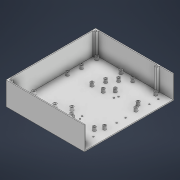
# Autodesk Inventor part: Grundplatte_vorne
Saved by Autodesk Inventor 2021 (Build 250183000, 183)
## iProperties
Created: 2021-01-26
Part Number: Grundplatte_vorne
Material: Generisch
Document SubType Name: Modeling
Designer: Ctroi
Density: 1 g/cm^3
Appearance: Vorgabe
Author: Ctroi
Autodesk Inventor part; units mm, degrees
ref_plane "YZ Plane" through (0, 0, 0) normal (1, 0, 0) x (0, 1, 0)
ref_plane "XZ Plane" through (0, 0, 0) normal (0, 1, 0) x (-1, 0, 0)
ref_plane "XY Plane" through (0, 0, 0) normal (0, 0, 1) x (1, 0, 0)
sketch "Skizze1" plane through (0, 0, 0) normal (0, 1, 0) x (-1, 0, 0)
  line L0 (0, -140) -> (0, 140) projected
  line L1 (-122.5, 0) -> (122.5, 0) projected
  line L2 (87.5, -100) -> (-87.5, -100)
  line L3 (-87.5, -100) -> (-87.5, 100)
  line L4 (-87.5, 100) -> (87.5, 100)
  line L5 (87.5, 100) -> (87.5, -100)
  point P0 (0, 0)
  dimension "d0" = 175
  dimension "d1" = 200
  constraints: 8 end point, 2 parallel, 1 horizontal, 1 perpendicular, 2 other
  measures "d0" distance of L3.end L4.end
  measures "d1" distance of L2.end L3.end
extrude "Extrusion1" add sketch "Skizze1" along normal blind 2
sketch "Skizze2" plane through (0, 2, 0) normal (0, 1, 0) x (1, 0, 0)
  circle A0 centre (70, 82.5) radius 1.6
  line L0 (87.5, -100) -> (87.5, 100) projected
  line L1 (87.5, 100) -> (-87.5, 100) projected
  circle A1 centre (70, 62.5) radius 1.6
  line L2 (122.5, 0) -> (-122.5, 0) projected
  circle A2 centre (70, -82.5) radius 1.6
  circle A3 centre (70, -62.5) radius 1.6
  point P0 (0, 0)
  dimension "d4" = 3.2
  dimension "d5" = 17.5
  dimension "d6" = 17.5
  dimension "d7" = 3.2
  dimension "d8" = 20
  dimension "d9" = 17.5
  constraints: 4 centre point, 2 symmetric about line, 2 other
  measures "d4" diameter of A0
  measures "d5" distance from line of L0 A0.centre
  measures "d6" distance from line of L1 A0.centre
  measures "d7" diameter of A1
  measures "d8" distance of A0.centre A1.centre
  measures "d9" distance from line of L0 A1.centre
extrude "Extrusion2" cut sketch "Skizze2" against normal up to surface (2 mm away)
sketch "Skizze4" plane through (0, 2, 0) normal (0, 1, 0) x (1, 0, 0)
  line L0 (-87.5, -100) -> (87.5, -100) projected
  line L1 (-87.5, 100) -> (-87.5, -100) projected
  line L2 (87.5, -100) -> (-87.5, -100)
  line L3 (-87.5, -100) -> (-87.5, -98)
  line L4 (-87.5, -98) -> (87.5, -98)
  line L5 (87.5, -98) -> (87.5, -100)
  line L6 (87.5, 100) -> (-87.5, 100) projected
  line L7 (87.5, 100) -> (-87.5, 100)
  line L8 (-87.5, 100) -> (-87.5, 98)
  line L9 (-87.5, 98) -> (87.5, 98)
  line L10 (87.5, 98) -> (87.5, 100)
  line L11 (87.5, -98) -> (51.5, -98)
  line L12 (51.5, -98) -> (51.5, -92)
  line L13 (51.5, -92) -> (57.5, -92)
  line L14 (87.5, 98) -> (51.5, 98)
  line L15 (51.5, 98) -> (51.5, 92)
  line L16 (51.5, 92) -> (57.5, 92)
  line L17 (-87.5, -98) -> (-85.5, -98)
  line L18 (-85.5, -98) -> (-85.5, 98)
  line L19 (-85.5, 98) -> (-87.5, 98)
  line L20 (-87.5, 98) -> (-87.5, -98)
  line L21 (-85.5, 98) -> (-79.5, 98)
  line L22 (-79.5, 98) -> (-79.5, 92)
  line L23 (-79.5, 92) -> (-85.5, 92)
  line L24 (-85.5, 92) -> (-85.5, 98)
  line L25 (-85.5, -98) -> (-79.5, -98)
  line L26 (-79.5, -98) -> (-79.5, -92)
  line L27 (-79.5, -92) -> (-85.5, -92)
  line L28 (-85.5, -92) -> (-85.5, -98)
  line L29 (57.5, -92) -> (57.5, -98)
  line L30 (87.5, -100) -> (87.5, 100) projected
  line L31 (57.5, 98) -> (57.5, 92)
  point P0 (0, 0)
  point P1 (-85.5, -92)
  point P2 (51.5, -98)
  point P3 (-87.5, 98)
  point P4 (-87.5, 100)
  dimension "d18" = 2
  dimension "d19" = 2
  dimension "d21" = 6
  dimension "d23" = 6
  dimension "d24" = 2
  dimension "d25" = 6
  dimension "d26" = 6
  dimension "d27" = 6
  dimension "d28" = 6
  dimension "d130" = 6
  dimension "d131" = 30
  dimension "d132" = 6
  dimension "d133" = 30
  constraints: 56 end point, 12 parallel, 9 perpendicular, 7 horizontal, 5 point on line
  measures "d18" distance of L2.end L3.end
  measures "d19" distance of L8.end L7.end
  measures "d21" distance of L11.end L12.end
  measures "d23" distance of L15.end L14.end
  measures "d24" distance of L19.end L18.end
  measures "d25" distance of L22.end L23.end
  measures "d26" distance of L21.end L22.end
  measures "d27" distance of L27.end L26.end
  measures "d28" distance of L26.end L25.end
  measures "d130" distance between parallel lines of L12 L29
  measures "d131" distance between parallel lines of L30 L29
  measures "d132" distance between parallel lines of L31 L15
  measures "d133" distance between parallel lines of L30 L31
extrude "Extrusion4" add sketch "Skizze4" along normal blind 50 contours L1 L4 L5 L0 | L1 L9 L18 L4 | L1 L6 L10 L9 | L18 L27 L26 L4 | L4 L12 L13 L29 | L9 L22 L23 L18 | L31 L16 L15 L9
sketch "Skizze5" plane through (0, 2, 0) normal (0, 1, 0) x (1, 0, 0)
  circle A0 centre (67.5, 35) radius 3.5
  circle A1 centre (67.5, -35) radius 3.5
  line L0 (-129.052, 0) -> (123.592, 0) projected
  line L1 (123.592, 0) -> (-129.052, 0) projected
  line L2 (87.5, -98) -> (87.5, 98) projected
  circle A2 centre (-5.5, -35) radius 3.5
  circle A3 centre (-5.5, 35) radius 3.5
  line L3 (87.5, 100) -> (-87.5, 100) projected
  circle A4 centre (-30, -48.325) radius 3.5
  circle A5 centre (-30, 34.225) radius 3.5
  circle A6 centre (-78.26, 27.875) radius 3.5
  circle A7 centre (-78.26, -47.055) radius 3.5
  line L4 (-87.5, 100) -> (-87.5, -100) projected
  line L5 (51.5, -98) -> (-79.5, -98) projected
  line L6 (-85.5, -92) -> (-85.5, 92) projected
  line L7 (0, 140) -> (0, -140) projected
  circle A8 centre (7.5, 49) radius 3.5
  circle A9 centre (7.5, 88) radius 3.5
  circle A10 centre (58.5, 49) radius 3.5
  circle A11 centre (58.5, 88) radius 3.5
  line L8 (-79.5, 98) -> (51.5, 98) projected
  circle A12 centre (7.5, -49) radius 3.5
  circle A13 centre (7.5, -88) radius 3.5
  circle A14 centre (58.5, -49) radius 3.5
  circle A15 centre (58.5, -88) radius 3.5
  circle A16 centre (-75.5, 56.5) radius 3.5
  circle A17 centre (-75.5, 90.5) radius 3.5
  circle A18 centre (-21.5, 56.5) radius 3.5
  circle A19 centre (-21.5, 90.5) radius 3.5
  circle A20 centre (-9, 73) radius 3.5
  circle A21 centre (-9, -73) radius 3.5
  point P0 (0, 0)
  point P1 (-75, 100)
  dimension "d31" = 7
  dimension "d32" = 7
  dimension "d35" = 20
  dimension "d36" = 20
  dimension "d37" = 7
  dimension "d38" = 73
  dimension "d40" = 7
  dimension "d42" = 73
  dimension "d68" = 70
  dimension "d69" = 70
  dimension "d70" = 35
  dimension "d73" = 65
  dimension "d74" = 7
  dimension "d75" = 7
  dimension "d83" = 7
  dimension "d86" = 7
  dimension "d136" = 48.26
  dimension "d137" = 74.93
  dimension "d138" = 48.26
  dimension "d139" = 82.55
  dimension "d142" = 30
  dimension "d143" = 30
  dimension "d144" = 34.225
  dimension "d145" = 47.055
  dimension "d148" = 7
  dimension "d149" = 7
  dimension "d150" = 7
  dimension "d151" = 7
  dimension "d152" = 10
  dimension "d153" = 10
  dimension "d154" = 39
  dimension "d155" = 39
  dimension "d156" = 51
  dimension "d157" = 51
  dimension "d161" = 7.5
  dimension "d163" = 7.5
  dimension "d177" = 7
  dimension "d178" = 7
  dimension "d179" = 7
  dimension "d180" = 7
  dimension "d181" = 10
  dimension "d182" = 10
  dimension "d183" = 7.5
  dimension "d184" = 34
  dimension "d185" = 7.5
  dimension "d186" = 34
  dimension "d187" = 54
  dimension "d188" = 54
  dimension "d193" = 7
  dimension "d194" = 25
  dimension "d195" = 9
  dimension "d196" = 7
  dimension "d197" = 25
  dimension "d198" = 9
  constraints: 22 centre point, 4 symmetric about line, 5 other
  measures "d31" diameter of A0
  measures "d32" diameter of A1
  measures "d35" distance from line of L2 A0.centre
  measures "d36" distance from line of L2 A1.centre
  measures "d37" diameter of A2
  measures "d38" distance of A1.centre A2.centre
  measures "d40" diameter of A3
  measures "d42" distance of A0.centre A3.centre
  measures "d68" distance of A0.centre A1.centre
  measures "d69" distance of A3.centre A2.centre
  measures "d70" distance from line of L0 A0.centre
  measures "d73" distance from line of L3 A3.centre
  measures "d74" diameter of A4
  measures "d75" diameter of A5
  measures "d83" diameter of A6
  measures "d86" diameter of A7
  measures "d136" horizontal distance of A4.centre A7.centre
  measures "d137" distance of A6.centre A7.centre
  measures "d138" horizontal distance of A5.centre A6.centre
  measures "d139" distance of A4.centre A5.centre
  measures "d142" distance from line of L7 A4.centre
  measures "d143" distance from line of L7 A5.centre
  measures "d144" distance from line of L1 A5.centre
  measures "d145" distance from line of L1 A7.centre
  measures "d148" diameter of A8
  measures "d149" diameter of A9
  measures "d150" diameter of A10
  measures "d151" diameter of A11
  measures "d152" distance from line of L8 A11.centre
  measures "d153" distance from line of L8 A9.centre
  measures "d154" distance of A9.centre A8.centre
  measures "d155" distance of A11.centre A10.centre
  measures "d156" distance of A11.centre A9.centre
  measures "d157" distance of A8.centre A10.centre
  measures "d161" distance from line of L7 A8.centre
  measures "d163" distance from line of L7 A9.centre
  measures "d177" diameter of A16
  measures "d178" diameter of A17
  measures "d179" diameter of A18
  measures "d180" diameter of A19
  measures "d181" distance from line of L6 A16.centre
  measures "d182" distance from line of L6 A17.centre
  measures "d183" distance from line of L8 A17.centre
  measures "d184" distance of A16.centre A17.centre
  measures "d185" distance from line of L8 A19.centre
  measures "d186" distance of A19.centre A18.centre
  measures "d187" distance of A17.centre A19.centre
  measures "d188" distance of A16.centre A18.centre
  measures "d193" diameter of A20
  measures "d194" distance from line of L8 A20.centre
  measures "d195" distance from line of L7 A20.centre
  measures "d196" diameter of A21
  measures "d197" distance from line of L5 A21.centre
  measures "d198" distance from line of L7 A21.centre
extrude "Extrusion5" add sketch "Skizze5" along normal blind 7 contours A0 | A1 | A2 | A3 | A4 | A5 | A6 | A7 | A8 | A9 | A10 | A11 | A12 | A13 | A14 | A15 | A16 | A17 | A18 | A19 | A20 | A21
sketch "Skizze6" plane through (-5.5, 9, -35) normal (0, 1, 0) x (1, 0, 0)
  circle A0 centre (0, 0) radius 2
  circle A1 centre (73, 0) radius 3.5 projected
  circle A2 centre (73, 0) radius 2
  circle A3 centre (0, -70) radius 2
  circle A4 centre (0, -70) radius 3.5 projected
  circle A5 centre (73, -70) radius 3.5 projected
  circle A6 centre (73, -70) radius 2
  circle A7 centre (-72.76, -82.055) radius 2
  circle A8 centre (-72.76, -82.055) radius 3.5 projected
  circle A9 centre (-24.5, -83.325) radius 2
  circle A10 centre (-24.5, -83.325) radius 3.5 projected
  circle A11 centre (-24.5, -0.775) radius 2
  circle A12 centre (-24.5, -0.775) radius 3.5 projected
  circle A13 centre (-72.76, -7.125) radius 2
  circle A14 centre (-72.76, -7.125) radius 3.5 projected
  circle A15 centre (13, -123) radius 3.5
  circle A16 centre (13, -123) radius 3.5 projected
  circle A17 centre (13, -123) radius 2
  circle A18 centre (13, -84) radius 3.5
  circle A19 centre (13, -84) radius 3.5 projected
  circle A20 centre (13, -84) radius 2
  circle A21 centre (64, -123) radius 2
  circle A22 centre (64, -123) radius 3.5 projected
  circle A23 centre (64, -123) radius 3.5
  circle A24 centre (64, -84) radius 3.5
  circle A25 centre (64, -84) radius 3.5 projected
  circle A26 centre (64, -84) radius 2
  line L0 (128, -35) -> (-117, -35) projected
  circle A27 centre (13, 53) radius 3.5
  circle A28 centre (13, 53) radius 2
  circle A29 centre (13, 14) radius 3.5
  circle A30 centre (13, 14) radius 2
  circle A31 centre (64, 53) radius 2
  circle A32 centre (64, 53) radius 3.5
  circle A33 centre (64, 14) radius 3.5
  circle A34 centre (64, 14) radius 2
  circle A35 centre (-70, 21.5) radius 3.5 projected
  circle A36 centre (-70, 55.5) radius 3.5 projected
  circle A37 centre (-16, 55.5) radius 3.5 projected
  circle A38 centre (-16, 21.5) radius 3.5 projected
  circle A39 centre (-70, 21.5) radius 2
  circle A40 centre (-70, 55.5) radius 3.5 projected
  circle A41 centre (-70, 55.5) radius 2
  circle A42 centre (-16, 21.5) radius 3.5 projected
  circle A43 centre (-16, 21.5) radius 2
  circle A44 centre (-16, 55.5) radius 3.5 projected
  circle A45 centre (-16, 55.5) radius 2
  circle A46 centre (-3.5, -108) radius 3.5 projected
  circle A47 centre (-3.5, 38) radius 3.5 projected
  circle A48 centre (-3.5, -108) radius 2
  circle A49 centre (-3.5, 38) radius 3.5 projected
  circle A50 centre (-3.5, 38) radius 2
  point P0 (-82, -78.8303)
  point P1 (-82, -84.6297)
  point P2 (-82, -3.9003)
  point P3 (-82, -9.6997)
  dimension "d45" = 4
  dimension "d46" = 4
  dimension "d47" = 4
  dimension "d48" = 0
  dimension "d49" = 4
  dimension "d50" = 73
  dimension "d51" = 70
  dimension "d96" = 4
  dimension "d97" = 0
  dimension "d98" = 0
  dimension "d99" = 4
  dimension "d100" = 0
  dimension "d101" = 0
  dimension "d102" = 4
  dimension "d103" = 0
  dimension "d104" = 4
  dimension "d105" = 0
  dimension "d164" = 7
  dimension "d165" = 0
  dimension "d166" = 0
  dimension "d167" = 4
  dimension "d168" = 7
  dimension "d169" = 0
  dimension "d170" = 4
  dimension "d171" = 4
  dimension "d172" = 0
  dimension "d173" = 7
  dimension "d174" = 7
  dimension "d176" = 4
  dimension "d189" = 4
  dimension "d190" = 4
  dimension "d191" = 4
  dimension "d192" = 4
  dimension "d199" = 4
  dimension "d200" = 4
  constraints: 30 centre point, 13 coincident, 8 symmetric about line, 10 other
  measures "d45" diameter of A0
  measures "d46" diameter of A2
  measures "d47" diameter of A3
  measures "d48" distance of A4.centre A3.centre
  measures "d49" diameter of A6
  measures "d50" distance of A2.centre A0.centre
  measures "d51" distance of A3.centre A0.centre
  measures "d96" diameter of A7
  measures "d97" distance of point (-72.76, -82.055) A7.centre
  measures "d98" distance of point (-72.76, -82.055) A7.centre
  measures "d99" diameter of A9
  measures "d100" distance of A10.centre A9.centre
  measures "d101" distance of A10.centre A9.centre
  measures "d102" diameter of A11
  measures "d103" distance of A12.centre A11.centre
  measures "d104" diameter of A13
  measures "d105" distance of point (-72.76, -7.125) A13.centre
  measures "d164" diameter of A15
  measures "d165" distance of A16.centre A15.centre
  measures "d166" distance of A16.centre A15.centre
  measures "d167" diameter of A17
  measures "d168" diameter of A18
  measures "d169" distance of A19.centre A18.centre
  measures "d170" diameter of A20
  measures "d171" diameter of A21
  measures "d172" distance of A22.centre A21.centre
  measures "d173" diameter of A23
  measures "d174" diameter of A24
  measures "d176" diameter of A26
  measures "d189" diameter of A39
  measures "d190" diameter of A41
  measures "d191" diameter of A43
  measures "d192" diameter of A45
  measures "d199" diameter of A48
  measures "d200" diameter of A50
extrude "Extrusion6" cut sketch "Skizze6" against normal blind 5 contours A0 | A2 | A3 | A6 | A7 | A9 | A11 | A13 | A17 | A20 | A21 | A26 | A28 | A30 | A31 | A34 | A39 | A41 | A43 | A45 | A48 | A50
sketch "Skizze7" plane through (0, 52, 0) normal (0, 1, 0) x (1, 0, 0)
  circle A0 centre (54.5, -95) radius 2
  circle A1 centre (-82.5, -95) radius 2
  circle A2 centre (-82.5, 95) radius 2
  circle A3 centre (54.5, 95) radius 2
  line L0 (51.5, 98) -> (51.5, 92) projected
  line L1 (51.5, 92) -> (57.5, 92) projected
  line L2 (51.5, -92) -> (51.5, -98) projected
  line L3 (57.5, -92) -> (51.5, -92) projected
  line L4 (-79.5, -98) -> (-79.5, -92) projected
  line L5 (-79.5, -92) -> (-85.5, -92) projected
  line L6 (-79.5, 92) -> (-79.5, 98) projected
  line L7 (-85.5, 92) -> (-79.5, 92) projected
  line L8 (57.5, -98) -> (57.5, -92) projected
  line L9 (57.5, 92) -> (57.5, 98) projected
  point P0 (0, 0)
  point P1 (75, -92)
  dimension "d54" = 4
  dimension "d55" = 4
  dimension "d56" = 4
  dimension "d57" = 4
  dimension "d59" = 3
  dimension "d61" = 3
  dimension "d62" = 3
  dimension "d63" = 3
  dimension "d64" = 3
  dimension "d65" = 3
  dimension "d146" = 3
  dimension "d147" = 3
  constraints: 4 centre point
  measures "d54" diameter of A0
  measures "d55" diameter of A1
  measures "d56" diameter of A2
  measures "d57" diameter of A3
  measures "d59" distance from line of L1 A3.centre
  measures "d61" distance from line of L3 A0.centre
  measures "d62" distance from line of L4 A1.centre
  measures "d63" distance from line of L5 A1.centre
  measures "d64" distance from line of L6 A2.centre
  measures "d65" distance from line of L7 A2.centre
  measures "d146" distance from line of L2 A0.centre
  measures "d147" distance from line of L0 A3.centre
extrude "Extrusion7" cut sketch "Skizze7" against normal blind 5
sketch "Skizze8" plane through (0, 2, 0) normal (0, 1, 0) x (1, 0, 0)
  circle A0 centre (69.5, 10) radius 1.6
  line L0 (122.5, 0) -> (-122.5, 0) projected
  line L1 (87.5, -98) -> (87.5, 98) projected
  circle A1 centre (69.5, -10) radius 1.6
  circle A2 centre (20.609, 42.961) radius 1.6
  circle A3 centre (17.873, 35.444) radius 1.6
  circle A4 centre (20.609, -42.961) radius 1.6
  circle A5 centre (17.873, -35.444) radius 1.6
  point P0 (0, 0)
  point P1 (75, -92)
  point P2 (75, 92)
  point P3 (87.5, 98)
  dimension "d119" = 3.2
  dimension "d120" = 18
  dimension "d121" = 10
  dimension "d122" = 3.2
  dimension "d123" = 3.2
  dimension "d124" = 66.891
  dimension "d125" = 69.627
  dimension "d126" = 42.961
  dimension "d127" = 35.444
  constraints: 6 centre point, 3 symmetric about line, 4 other
  measures "d119" diameter of A0
  measures "d121" distance from line of L0 A0.centre
  measures "d122" diameter of A2
  measures "d123" diameter of A3
  measures "d126" distance from line of L0 A2.centre
  measures "d127" distance from line of L0 A3.centre
extrude "Extrusion8" cut sketch "Skizze8" against normal up to surface (2 mm away)
equation "\"d43\" = d83"
